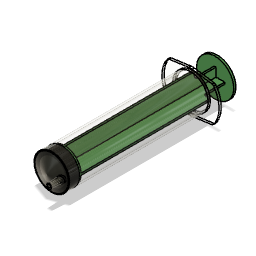
Syringe 50ml v10 (Autodesk Fusion 360 design; units mm, degrees)
Autodesk Fusion 360 part; units mm, degrees
sketch "Skizze3" plane through (0, 0, 0) normal (1, 0, 0) x (0, 0, -1)
  line L0 (0, 0) -> (0, 14.5) construction
  line L1 (0, 14.5) -> (-116, 14.4367)
  line L2 (0, 14.5) -> (91.9999, 14.5) construction
  line L3 (-116, 14.4367) -> (-71.8483, 14.4367) construction
  line L4 (0, 0) -> (-121.2545, 0) construction
  line L5 (-116, 14.4367) -> (-121.2545, 0)
  line L6 (-116, 14.4367) -> (-73.1003, 14.4367) construction
  line L7 (0, 14.5) -> (0.0007, 13.3)
  line L8 (0.0007, 13.3) -> (-115.0776, 13.2372)
  line L9 (-115.0776, 13.2372) -> (-119.8956, 0)
  line L10 (-109.39, 28.8637) -> (-110.59, 29.3004) construction
  line L11 (-121.2545, 0) -> (-119.8956, 0)
  dimension "d19" = 14.5
  dimension "d20" = 180.031
  dimension "d21" = 116
  dimension "d24" = 110
  dimension "d25" = 1.2
  dimension "d26" = 1.2
  constraint coincident L0.start L4.start
  constraint vertical L0
  constraint horizontal L2
  constraint horizontal L3
  constraint horizontal L4
  constraint horizontal L6
  constraint coincident L4 L5.end
  constraint coincident L4.end L5.end
  constraint perpendicular L1 L7
  constraint parallel L1 L8
  constraint parallel L5 L9
  constraint coincident L4 L9.end
  constraint coincident L9 L10.start
  constraint coincident L5 L10.end
  constraint perpendicular L5 L10
  measures "d19" distance of L0.start L0.end
  measures "d21" distance of L0.end L1.end
  measures "d24" angle of L5 L6
  measures "d25" distance of L0.end L7.end
  measures "d26" horizontal distance of L10.start L10.end
revolve "Drehen1" add sketch "Skizze3" angle 360 about axis through (0, 0, 0) along (0, 0, 1) makes body 1
sketch "Skizze4" plane through (0, 0, 0) normal (0, 0, 1) x (1, 0, 0)
  circle A0 centre (0, 0) radius 15.3
  dimension "d29" = 30.6
  constraint coincident A0.centre origin
  measures "d29" diameter of A0
extrude "Extrusion3" add sketch "Skizze4" against normal blind 1.75 from surface at -18.5 separate body makes body 2
sketch "Skizze6" plane through (0, 0, -20.25) normal (0, 0, -1) x (-1, 0, 0)
  circle A0 centre (0, 0) radius 15.3 construction
  circle A1 centre (0, 0) radius 15.3
  line L0 (-0.275, 15.3) -> (0.275, 15.3)
  line L1 (0.275, 15.3) -> (0.275, -15.3)
  line L2 (0.275, -15.3) -> (-0.275, -15.3)
  line L3 (-0.275, -15.3) -> (-0.275, 15.3)
  line L4 (-0.275, 0) -> (0.275, 0) construction
  line L5 (-13.775, -15.3) -> (-13.775, 15.3)
  line L6 (-13.225, 15.3) -> (-13.225, -15.3)
  line L7 (-13.775, 15.3) -> (-13.225, 15.3)
  line L8 (-13.225, -15.3) -> (-13.775, -15.3)
  line L9 (-12.275, -15.3) -> (-12.275, 15.3)
  line L10 (-11.725, 15.3) -> (-11.725, -15.3)
  line L11 (-12.275, 15.3) -> (-11.725, 15.3)
  line L12 (-11.725, -15.3) -> (-12.275, -15.3)
  line L13 (-10.775, -15.3) -> (-10.775, 15.3)
  line L14 (-10.225, 15.3) -> (-10.225, -15.3)
  line L15 (-10.775, 15.3) -> (-10.225, 15.3)
  line L16 (-10.225, -15.3) -> (-10.775, -15.3)
  line L17 (-9.275, -15.3) -> (-9.275, 15.3)
  line L18 (-8.725, 15.3) -> (-8.725, -15.3)
  line L19 (-9.275, 15.3) -> (-8.725, 15.3)
  line L20 (-8.725, -15.3) -> (-9.275, -15.3)
  line L21 (-7.775, -15.3) -> (-7.775, 15.3)
  line L22 (-7.225, 15.3) -> (-7.225, -15.3)
  line L23 (-7.775, 15.3) -> (-7.225, 15.3)
  line L24 (-7.225, -15.3) -> (-7.775, -15.3)
  line L25 (-6.275, -15.3) -> (-6.275, 15.3)
  line L26 (-5.725, 15.3) -> (-5.725, -15.3)
  line L27 (-6.275, 15.3) -> (-5.725, 15.3)
  line L28 (-5.725, -15.3) -> (-6.275, -15.3)
  line L29 (-4.775, -15.3) -> (-4.775, 15.3)
  line L30 (-4.225, 15.3) -> (-4.225, -15.3)
  line L31 (-4.775, 15.3) -> (-4.225, 15.3)
  line L32 (-4.225, -15.3) -> (-4.775, -15.3)
  line L33 (-3.275, -15.3) -> (-3.275, 15.3)
  line L34 (-2.725, 15.3) -> (-2.725, -15.3)
  line L35 (-3.275, 15.3) -> (-2.725, 15.3)
  line L36 (-2.725, -15.3) -> (-3.275, -15.3)
  line L37 (-1.775, -15.3) -> (-1.775, 15.3)
  line L38 (-1.225, 15.3) -> (-1.225, -15.3)
  line L39 (-1.775, 15.3) -> (-1.225, 15.3)
  line L40 (-1.225, -15.3) -> (-1.775, -15.3)
  line L41 (1.225, -15.3) -> (1.225, 15.3)
  line L42 (1.775, 15.3) -> (1.775, -15.3)
  line L43 (1.225, 15.3) -> (1.775, 15.3)
  line L44 (1.775, -15.3) -> (1.225, -15.3)
  line L45 (2.725, -15.3) -> (2.725, 15.3)
  line L46 (3.275, 15.3) -> (3.275, -15.3)
  line L47 (2.725, 15.3) -> (3.275, 15.3)
  line L48 (3.275, -15.3) -> (2.725, -15.3)
  line L49 (4.225, -15.3) -> (4.225, 15.3)
  line L50 (4.775, 15.3) -> (4.775, -15.3)
  line L51 (4.225, 15.3) -> (4.775, 15.3)
  line L52 (4.775, -15.3) -> (4.225, -15.3)
  line L53 (5.725, -15.3) -> (5.725, 15.3)
  line L54 (6.275, 15.3) -> (6.275, -15.3)
  line L55 (5.725, 15.3) -> (6.275, 15.3)
  line L56 (6.275, -15.3) -> (5.725, -15.3)
  line L57 (7.225, -15.3) -> (7.225, 15.3)
  line L58 (7.775, 15.3) -> (7.775, -15.3)
  line L59 (7.225, 15.3) -> (7.775, 15.3)
  line L60 (7.775, -15.3) -> (7.225, -15.3)
  line L61 (8.725, -15.3) -> (8.725, 15.3)
  line L62 (9.275, 15.3) -> (9.275, -15.3)
  line L63 (8.725, 15.3) -> (9.275, 15.3)
  line L64 (9.275, -15.3) -> (8.725, -15.3)
  line L65 (10.225, -15.3) -> (10.225, 15.3)
  line L66 (10.775, 15.3) -> (10.775, -15.3)
  line L67 (10.225, 15.3) -> (10.775, 15.3)
  line L68 (10.775, -15.3) -> (10.225, -15.3)
  line L69 (11.725, -15.3) -> (11.725, 15.3)
  line L70 (12.275, 15.3) -> (12.275, -15.3)
  line L71 (11.725, 15.3) -> (12.275, 15.3)
  line L72 (12.275, -15.3) -> (11.725, -15.3)
  line L73 (13.225, -15.3) -> (13.225, 15.3)
  line L74 (13.775, 15.3) -> (13.775, -15.3)
  line L75 (13.225, 15.3) -> (13.775, 15.3)
  line L76 (13.775, -15.3) -> (13.225, -15.3)
  line L77 (14.725, -15.3) -> (14.725, 15.3)
  line L78 (15.275, 15.3) -> (15.275, -15.3)
  line L79 (14.725, 15.3) -> (15.275, 15.3)
  line L80 (15.275, -15.3) -> (14.725, -15.3)
  dimension "d35" = 0.55
  dimension "d36" = 30.6
  dimension "d40" = 1.5
  dimension "d41" = 0
  constraint horizontal L0
  constraint vertical L1
  constraint horizontal L2
  constraint vertical L3
  constraint midpoint L3 L4.start
  constraint midpoint L1 L4.end
  constraint midpoint L4 A0.centre
  constraint coincident A0.centre A1.centre
  measures "d35" distance of L0.start L0.end
  measures "d36" distance of L0.start L2.end
extrude "Extrusion4" add sketch "Skizze6" along normal blind 0.2 contours A1 L73 L74 | A1 L69 L70 | A1 L65 L66 | A1 L61 L62 | A1 L57 L58 | A1 L53 L54 | A1 L49 L50 | A1 L45 L46 | A1 L41 L42 | A1 L1 L3 | A1 L37 L38 | A1 L33 L34 | A1 L29 L30 | A1 L25 L26 | A1 L21 L22 | A1 L17 L18 | A1 L13 L14 | A1 L9 L10 | A1 L5 L6 bodies 2
sketch "Plunger serration bottom removal" plane through (0, 0, -20.25) normal (0, 0, -1) x (-1, 0, 0)
  line L0 (-0.275, -15.2975) -> (-0.275, 15.2975)
  arc A0 (-6.275, 13.954) -> (-7.225, 13.4866) centre (0, 0) ccw
  line L1 (-7.225, 13.4866) -> (-7.225, -13.4866)
  arc A1 (-7.225, -13.4866) -> (-6.275, -13.954) centre (0, 0) ccw
  circle A2 centre (0, 0) radius 13.77
  circle A3 centre (0, 0) radius 15.3
  line L2 (-6.275, -13.954) -> (-6.275, 13.954)
  arc A4 (-0.275, 15.2975) -> (-1.225, 15.2509) centre (0, 0) ccw
  line L3 (-1.225, 15.2509) -> (-1.225, -15.2509)
  arc A5 (-1.225, -15.2509) -> (-0.275, -15.2975) centre (0, 0) ccw
  dimension "d98" = 27.54
  dimension "d99" = 30.6
  constraint coincident A0.centre A1.centre
  constraint concentric A2 A3
  measures "d98" diameter of A2
  measures "d99" diameter of A3
extrude "Extrusion9" cut sketch "Plunger serration bottom removal" along normal blind 0.2 draft 70 contours L0 A2 A3 L3 A5 | L0 A2 A3 | A2 A3 L2 L3 | L0 A2 A3 A4 L3 | L1 A1 A2 A3 L2 | A2 A3 L2 L3 | L1 A2 A3 | A0 L1 A2 A3 L2 bodies 2
sketch "Skizze7" plane through (0, 0, -18.5) normal (0, 0, 1) x (1, 0, 0)
  circle A0 centre (0, 0) radius 15.3
  line L0 (-0.75, 15.2816) -> (0.75, 15.2816)
  line L1 (0.75, 15.2816) -> (0.75, -15.2816)
  line L2 (0.75, -15.2816) -> (-0.75, -15.2816)
  line L3 (-0.75, -15.2816) -> (-0.75, 15.2816)
  circle A1 centre (0, 0) radius 15.3
  line L4 (15.2816, 0.75) -> (-15.2816, 0.75)
  line L5 (-15.2816, 0.75) -> (-15.2816, -0.75)
  line L6 (-15.2816, -0.75) -> (15.2816, -0.75)
  line L7 (15.2816, -0.75) -> (15.2816, 0.75)
  line L8 (13.675, 0.75) -> (13.675, -0.75)
  line L9 (13.675, 0) -> (0, 0) construction
  line L10 (-0.75, 13.675) -> (0.75, 13.675)
  line L11 (-13.675, -0.75) -> (-13.675, 0.75)
  line L12 (0.75, -13.675) -> (-0.75, -13.675)
  point P0 (-0.75, 15.2816)
  point P1 (0.75, 15.2816)
  dimension "d46" = 1.5
  dimension "d48" = 1.5
  dimension "d92" = 13.675
  dimension "d94" = 360
  constraint horizontal L0
  constraint vertical L1
  constraint horizontal L2
  constraint vertical L3
  constraint coincident P0 L0.start
  constraint coincident P1 L0.end
  constraint coincident P0 A1
  constraint coincident P1 A1
  constraint coincident L2.end A1
  constraint horizontal L4
  constraint vertical L5
  constraint horizontal L6
  constraint vertical L7
  constraint coincident A1 L4.start
  constraint coincident A1 L5.end
  constraint coincident A1 L4.end
  constraint coincident L4 L8.start
  constraint coincident L6 L8.end
  constraint perpendicular L6 L8
  constraint midpoint L8 L9.start
  constraint coincident A0.centre A1.centre
  constraint perpendicular L3 L9
  measures "d46" distance of P0 P1
  measures "d48" distance of L4.start L6.end
  measures "d92" distance of L9.start A0.centre
extrude "Extrusion5" add sketch "Skizze7" along normal blind 124 contours L1 L4 L6 L8 | L1 L3 L4 L10 | L1 L3 L4 L6 | L1 L3 L6 L12 | L3 L4 L6 L11 bodies 2
sketch "Skizze8" plane through (0, 0, 105.5) normal (0, 0, 1) x (1, 0, 0)
  line L0 (0.75, -0.75) -> (13.675, -0.75)
  line L1 (13.675, 0.75) -> (0.75, 0.75)
  line L2 (0.75, 0.75) -> (0.75, 13.675)
  line L3 (-0.75, 13.675) -> (-0.75, 0.75)
  line L4 (-0.75, 0.75) -> (-13.675, 0.75)
  line L5 (-13.675, -0.75) -> (-0.75, -0.75)
  line L6 (-0.75, -0.75) -> (-0.75, -13.675)
  line L7 (0.75, -13.675) -> (0.75, -0.75)
  circle A0 centre (0, 0) radius 15.3
  circle A1 centre (0, 0) radius 14.1375
  line L8 (13.675, -0.75) -> (13.675, 0.75)
  line L9 (0.75, 13.675) -> (-0.75, 13.675)
  line L10 (-13.675, 0.75) -> (-13.675, -0.75)
  line L11 (-0.75, -13.675) -> (0.75, -13.675)
  dimension "d55" = 28.275
  constraint concentric A0 A1
  measures "d55" diameter of A1
extrude "Extrusion6" add sketch "Skizze8" along normal blind 1.75 contours L0 L1 L2 L3 L4 L5 L6 L7 L8 L9 L10 L11 | A1 bodies 2
sketch "Skizze9" plane through (0, 0, 107.25) normal (0, 0, 1) x (1, 0, 0)
  circle A0 centre (0, 0) radius 14.5
  circle A1 centre (0, 0) radius 14.1375
  dimension "d54" = 29
  measures "d54" diameter of A0
extrude "Extrusion7" add sketch "Skizze9" along normal blind 8.75 separate body contours A1 makes body 3
fillet "Abrundung1" radius 0.5 1 edges at (-13.1808, -5.1123, 116) on bodies 3
sketch "Skizze10" plane through (0, 0, 0) normal (0, 1, 0) x (1, 0, 0)
  line L0 (-15.3, 18.5) -> (15.3, 18.5)
  line L1 (13.3, 0.0007) -> (-13.3, 0.0007)
  line L2 (13.2372, -115.0776) -> (-13.2372, -115.0776)
  line L3 (0, -115.0776) -> (13.775, -115.0776)
  line L4 (-15.3, 18.5) -> (15.3, 18.5)
  line L5 (13.2372, -115.0776) -> (13.775, -115.0776)
  line L6 (13.2372, -115.0776) -> (14.2372, -115.0776)
  line L7 (15.3, -116.4995) -> (15.3, 18.5)
  line L8 (7.9, 0.5) -> (7.9, 18.5)
  line L9 (15.3, -116.4995) -> (13.675, -116.4995)
  line L10 (13.675, 0.5) -> (13.675, -116.4995)
  line L11 (0, 0) -> (0, 9) construction
  line L12 (13.675, 0.5) -> (7.9, 0.5)
  line L13 (0, 9) -> (7.9, 9) construction
  line L14 (0, 0) -> (0, -5.4695) construction
  line L15 (0, -5.4695) -> (13.675, -5.4695) construction
  circle A0 centre (10.7875, 3.3875) radius 2.8875
  circle A1 centre (10.7875, -2.3875) radius 2.8875
  point P0 (0, 18.5)
  point P1 (7.9, 18.5)
  point P2 (-15.3, 18.5)
  dimension "d61" = 13.775
  dimension "d64" = 1
  dimension "d88" = 18
  dimension "d102" = 7.9
  dimension "d103" = 13.675
  dimension "d104" = 2.8875
  constraint midpoint L0 P0
  constraint midpoint L2 L3.start
  constraint parallel L2 L3
  constraint coincident L2.start L5.start
  constraint horizontal L6
  constraint coincident L0.end L4.end
  constraint coincident L4 P1
  constraint vertical L8
  constraint perpendicular L7 L9
  constraint perpendicular L9 L10
  constraint coincident P1 L8
  constraint vertical L7
  constraint horizontal L12
  constraint coincident L8 L13.end
  constraint perpendicular L8 L13
  constraint coincident L11.start L14.start
  constraint perpendicular L1 L14
  constraint coincident L10 L15.end
  constraint perpendicular L10 L15
  constraint tangent L8 A0
  constraint tangent L12 A0
  constraint symmetric L12 A0 A1
  measures "d61" distance of L3.start L3.end
  measures "d64" distance of L2.start L6.end
  measures "d88" distance of L8.start P1
  measures "d102" distance of L11.end L13.end
  measures "d103" distance of L14.end L15.end
  measures "d104" radius of A0
revolve "Drehen2" cut sketch "Skizze10" angle 360 about axis through (0, 0, 1.75) along (0, 0, 1) contours L0 L4 L7 L8 L9 L10 L12 A0 | A0 | L10 L12 A1 bodies 2
sketch "Skizze11" plane through (0, 0, 0) normal (0, 0, 1) x (1, 0, 0)
  circle A0 centre (0, 0) radius 13.3
  line L0 (0, 17) -> (23.5, 13.6973)
  line L1 (0, 10.5) -> (12.2678, 10.5) construction
  line L2 (0, 0) -> (23.5, 0) construction
  line L3 (23.5, 0) -> (23.5, 17) construction
  line L4 (0, 0) -> (0, 17) construction
  line L5 (0, -17) -> (23.5, -13.6973)
  line L6 (0, 17) -> (-23.5, 13.6973)
  line L7 (0, -17) -> (-23.5, -13.6973)
  line L8 (23.5, 13.6973) -> (23.5, -13.6973)
  line L9 (-23.5, 13.6973) -> (-23.5, -13.6973)
  circle A1 centre (0, 0) radius 23.5
  circle A2 centre (0, 0) radius 14.5
  dimension "d65" = 8
  dimension "d67" = 23.5
  dimension "d69" = 17
  dimension "d96" = 29
  constraint horizontal L1
  constraint coincident A0.centre L2.start
  constraint horizontal L2
  constraint perpendicular L2 L3
  constraint coincident L0.end L3
  constraint perpendicular L2 L4
  constraint coincident L0.start L4.end
  constraint symmetric L0.end L2 L5.end
  constraint symmetric L2 L0.start L5.start
  constraint symmetric L0.end L4 L6.end
  constraint symmetric L0.start L4 L6.start
  constraint symmetric L4 L5.start L7.start
  constraint symmetric L4 L5.end L7.end
  constraint concentric A0 A1
  constraint tangent L9 A1
  constraint concentric A0 A2
  measures "d65" angle of L0 L1
  measures "d67" distance of A0.centre L2.end
  measures "d69" distance of A0.centre L0.start
  measures "d96" diameter of A2
extrude "Extrusion8" add sketch "Skizze11" along normal blind 1.8 contours L0 L5 L6 L7 A1 bodies 1 2 3
fillet "Abrundung2" radius 10 2 edges at (0, 17, 0.9) (0, -17, 0.9) on bodies 1
fillet "Abrundung2" radius 2 4 edges at (18.5799, 14.3888, 0.9) (-18.5799, 14.3888, 0.9) (-18.5799, -14.3888, 0.9) (18.5799, -14.3888, 0.9) on bodies 1
sketch "Skizze14" plane through (0, 0, 0) normal (0, 1, 0) x (1, 0, 0)
  line L0 (13.2372, -115.0776) -> (-13.2372, -115.0776)
  line L1 (0, -115.0776) -> (9, -115.0776) construction
  line L2 (9, -115.0776) -> (9, -127.0776)
  line L3 (7, -127.0776) -> (6.2787, -115.0776)
  line L4 (7, -127.0776) -> (9.6268, -127.0776) construction
  line L5 (9, -127.0776) -> (7, -127.0776) construction
  line L6 (7.85, -127.0776) -> (7.85, -115.0776)
  line L7 (7.85, -115.0776) -> (9, -115.0776) construction
  line L8 (7.85, -127.0776) -> (7, -127.0776)
  line L9 (9, -115.0776) -> (6.5, -115.0776)
  line L10 (6.5, -115.0776) -> (6.5, -117.0776)
  line L11 (6.5, -117.0776) -> (9, -117.0776)
  line L12 (9, -117.0776) -> (9, -115.0776)
  dimension "d75" = 9
  dimension "d77" = 93.44
  dimension "d78" = 12
  dimension "d79" = 2
  dimension "d80" = 1.15
  dimension "d81" = 2.5
  dimension "d82" = 2
  constraint midpoint L0 L1.start
  constraint parallel L0 L1
  constraint perpendicular L1 L2
  constraint horizontal L4
  constraint coincident L1 L3.end
  constraint perpendicular L2 L5
  constraint coincident L3.start L5
  constraint vertical L6
  constraint coincident L4 L6.start
  constraint coincident L1 L6.end
  constraint horizontal L9
  constraint vertical L10
  constraint horizontal L11
  constraint vertical L12
  measures "d75" distance of L1.start L1.end
  measures "d77" angle of L3 L4
  measures "d78" distance of L1.end L2.end
  measures "d79" distance of L2.end L3.start
  measures "d80" distance of L1.end L6.end
  measures "d81" distance of L1.end L9.end
  measures "d82" distance of L1.end L11.end
revolve "Drehen3" add sketch "Skizze14" angle 360 about axis through (9, 0, 115.0776) along (0, 0, 1) bodies 1
equation "BackOuterDiameter = 31.4 mm"
equation "BackInnerDiameter = 29 mm"
equation "BodyDraftAngle = 0.03125 deg"
equation "BodyLength = 116 mm" comment "Excluding flange"
equation "FlangeDepth = 1.8 mm"
equation "PlungerCrossWidth = 1.5 mm"
equation "PlungerBottomDepth = 1.75 mm" comment "Also lengthof connector to rubber plunger"
equation "PlungerSerrationDepth = 0.2 mm"
equation "PlungerRubberPusherLength = 8.75 mm"
equation "PlungerExtraLength = 19 mm" comment "When fully inserted"
equation "d19 = BackInnerDiameter / 2"
equation "d20 = 180 deg + BodyDraftAngle"
equation "d21 = BodyLength"
equation "BodyFrontDraftAngle = 20 deg"
equation "d24 = 90 deg + BodyFrontDraftAngle"
equation "d25 = ( BackOuterDiameter - BackInnerDiameter ) / 2"
equation "d26 = ( BackOuterDiameter - BackInnerDiameter ) / 2"
equation "PlungerBottomDiameter = 30.6 mm"
equation "d29 = PlungerBottomDiameter"
equation "BodyFlangeAngle = 8 deg"
equation "d31 = -PlungerBottomDepth"
equation "PlungerSerrationDistance = 1.5 mm"
equation "PlungerSerrationWidth = 0.55 mm"
equation "d35 = PlungerSerrationWidth"
equation "d36 = PlungerBottomDiameter"
equation "NumSerrations = floor(PlungerBottomDiameter / PlungerSerrationDistance)"
equation "d38 = NumSerrations"
equation "d40 = PlungerSerrationDistance"
equation "d42 = PlungerSerrationDepth"
equation "d44 = -RetractedPlungerOffsetFromBody"
equation "RetractedPlungerOffsetFromBody = 18.5 mm"
equation "d46 = PlungerCrossWidth"
equation "d48 = PlungerCrossWidth"
equation "PlungerCrossLength = BodyLength + RetractedPlungerOffsetFromBody - PlungerRubberPusherLength - PlungerBottomDepth"
equation "d50 = PlungerCrossLength"
equation "d52 = PlungerBottomDepth"
equation "d54 = BackInnerDiameter"
equation "d55 = BackInnerDiameter * 0.975"
equation "d56 = PlungerRubberPusherLength"
equation "d61 = PlungerCrossDiameter / 2"
equation "PlungerCrossDiameter = 0.95 * BackInnerDiameter"
equation "d65 = BodyFlangeAngle"
equation "BodyFlangeWidth = 47 mm" comment "Width of the flange at the widest point"
equation "d67 = BodyFlangeWidth / 2"
equation "BodyFlangeHeight = 34 mm" comment "Width of the flange at the narrowest point"
equation "d69 = BodyFlangeHeight / 2"
equation "d70 = FlangeDepth"
equation "LuerOffsetFromCenter = 9 mm" comment "If the Luer connector is in the center, set this to 0"
equation "d75 = LuerOffsetFromCenter"
equation "d77 = 90 deg + 3.44 deg"
equation "d80 = ( 2.3 / 2 ) * 1 mm"
equation "PlungerCrossMinWidth = 15.8 mm"
equation "PlungerCrossMaxWidth = 27.35 mm"
equation "PlungerCrossMinWidthLength = 18 mm"
equation "d88 = PlungerCrossMinWidthLength"
equation "d92 = PlungerCrossMaxWidth / 2"
equation "d96 = BackInnerDiameter"
equation "d98 = 0.9 * PlungerBottomDiameter"
equation "d99 = PlungerBottomDiameter"
equation "d100 = PlungerSerrationDepth"
equation "d102 = PlungerCrossMinWidth / 2"
equation "d103 = PlungerCrossMaxWidth / 2"
equation "d104 = ( PlungerCrossMaxWidth - PlungerCrossMinWidth ) / 4"
named bodies: "Body", "Plunger", "Pusher"
